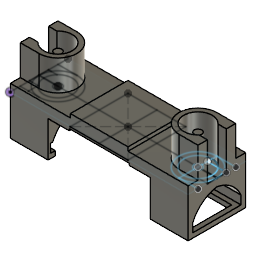
hexbug_cage_final (Autodesk Fusion 360 design; units mm, degrees)
Autodesk Fusion 360 part; units mm, degrees
note: some values were not read from the file. Set by a fixed rule: which sketch regions a step uses.
sketch "Sketch1" plane through (0, 0, 0) normal (0, 0, 1) x (1, 0, 0)
  line L0 (0, 0) -> (46.99, 0)
  line L1 (46.99, 0) -> (46.99, 15.24)
  line L2 (46.99, 15.24) -> (0, 15.24)
  line L3 (0, 15.24) -> (0, 0)
  line L4 (0, 0) -> (0, 1.25)
  line L5 (0, 1.25) -> (46.99, 1.25)
  line L6 (0, 15.24) -> (0, 13.99)
  line L7 (0, 13.99) -> (46.99, 13.99)
  dimension "d1" = 46.99
  dimension "d2" = 15.24
  dimension "d3" = 1.25
  dimension "d4" = 1.25
  constraint horizontal L0
  constraint vertical L1
  constraint horizontal L2
  constraint vertical L3
  constraint coincident L0.start L3.end
  constraint perpendicular L0 L4
  constraint coincident L1 L5.end
  constraint perpendicular L1 L5
  constraint perpendicular L2 L6
  constraint coincident L1 L7.end
  constraint perpendicular L1 L7
  measures "d1" distance of L0.start L0.end
  measures "d2" distance of L0.start L2.end
  measures "d3" distance of L0.start L4.end
  measures "d4" distance of L2.end L6.end
extrude "Extrude1" add sketch "Sketch1" along normal blind 2.27 contours L0 L1 L3 L4 L5 | L1 L2 L3 L6 L7 makes body 1 at (15.6633, 1.25, 0.7567) makes body 2 at (31.3267, 15.24, 0.7567)
sketch "Sketch2" plane through (0, 0, 2.27) normal (0, 0, 1) x (-1, 0, 0)
  line L0 (0, -13.99) -> (-46.99, -13.99)
  line L1 (-46.99, -13.99) -> (-46.99, -15.24)
  line L2 (-46.99, -15.24) -> (0, -15.24)
  line L3 (0, -15.24) -> (0, -13.99)
  line L4 (0, 0) -> (-46.99, 0)
  line L5 (-46.99, 0) -> (-46.99, -15.24)
  line L6 (-46.99, -15.24) -> (0, -15.24)
  line L7 (0, -15.24) -> (0, 0)
  constraint horizontal L4
  constraint vertical L5
  constraint horizontal L6
  constraint vertical L7
  constraint coincident L1.end L2.start
  constraint coincident L4.start L7.end
extrude "Extrude2" add sketch "Sketch2" along normal blind 7.08 contours L0 L4 L5 L7 bodies 1 2
extrude "Extrude3" add 1 faces at (15.6633, 14.8233, 2.27) along direction (0, 0, 1) blind 7.08 on bodies 1 bodies 1
sketch "Sketch3" plane through (0, 0, 0) normal (-1, 0, 0) x (0, -1, 0)
  line L0 (-15.24, 0) -> (-13.99, 0)
  line L1 (-13.99, 0) -> (-13.99, 2.27)
  line L2 (-13.99, 2.27) -> (-1.25, 2.27)
  line L3 (-1.25, 2.27) -> (-1.25, 0)
  line L4 (-1.25, 0) -> (0, 0)
  line L5 (0, 0) -> (0, 9.35)
  line L6 (0, 9.35) -> (-15.24, 9.35)
  line L7 (-15.24, 9.35) -> (-15.24, 0)
  line L8 (-15.24, 2.27) -> (-7.62, 2.27)
  line L9 (-7.62, 2.27) -> (-7.62, 7.35)
  line L10 (-7.62, 7.35) -> (-1.25, 2.27)
  line L11 (-7.62, 7.35) -> (-13.99, 2.27)
  line L12 (-4.435, 4.81) -> (-4.435, 7.35)
  line L13 (-4.435, 7.35) -> (-10.805, 7.35)
  line L14 (-10.805, 7.35) -> (-10.805, 4.81)
  arc A0 (-7.62, 7.35) -> (-13.99, 2.27) centre (-6.1125, -1.0741) ccw
  arc A1 (-1.25, 2.27) -> (-7.62, 7.35) centre (-9.128, -1.0747) ccw
  dimension "d11" = 5.08
  constraint coincident L7 L8.start
  constraint midpoint L2 L8.end
  constraint perpendicular L5 L8
  constraint perpendicular L2 L9
  constraint coincident L2.end L3.start
  constraint coincident L1.end L2.start
  constraint midpoint L10 L12.start
  constraint vertical L12
  constraint perpendicular L9 L13
  constraint midpoint L11 L14.end
  constraint perpendicular L13 L14
  measures "d11" distance of L8.end L9.end
extrude "Extrude4" cut sketch "Sketch3" against normal blind 60 contours L2 L8 L9 L11 | L11 L14 A0 | L2 L9 L10 | L11 L14 A0 | L10 L12 A1 | L10 L12 A1 bodies 1
sketch "Sketch4" plane through (0, 0, 9.35) normal (0, 0, 1) x (-1, 0, 0)
  line L0 (0, 0) -> (-46.99, 0)
  line L1 (-46.99, 0) -> (-46.99, -15.24)
  line L2 (-46.99, -15.24) -> (0, -15.24)
  line L3 (0, -15.24) -> (0, 0)
  line L4 (-46.99, -7.62) -> (0, -7.62)
  line L5 (0, 0) -> (0, -15.24)
  line L6 (0, -7.62) -> (-5, -7.62)
  circle A0 centre (-5, -7.62) radius 1
  line L7 (-46.99, -7.62) -> (-41.99, -7.62)
  circle A1 centre (-41.99, -7.62) radius 1
  line L8 (-41.99, -7.62) -> (-41.99, -8.62)
  line L9 (-41.99, -7.62) -> (-41.99, -6.62)
  circle A2 centre (-41.99, -7.62) radius 5
  line L10 (-41.99, -10.12) -> (-46.99, -10.12)
  circle A3 centre (-41.99, -7.62) radius 3.75
  circle A4 centre (-5, -7.62) radius 3.75
  circle A5 centre (-5, -7.62) radius 5
  line L11 (-23.495, -7.62) -> (-23.495, -15.24)
  line L12 (-23.495, -7.62) -> (-23.495, 0)
  line L13 (-15.875, -15.24) -> (-31.115, -15.24)
  line L14 (-31.115, -15.24) -> (-31.115, 0)
  line L15 (-31.115, 0) -> (-15.875, 0)
  line L16 (-15.875, 0) -> (-15.875, -15.24)
  line L17 (-15.875, -15.24) -> (-31.115, 0) construction
  line L18 (-31.115, -15.24) -> (-15.875, 0) construction
  line L19 (0, -7.62) -> (0, -5.12)
  line L20 (0, -5.12) -> (-0.6699, -5.12)
  line L21 (0, -7.62) -> (0, -10.12)
  line L22 (0, -10.12) -> (-0.6699, -10.12)
  line L23 (0, -10.12) -> (-2.2049, -10.12)
  line L24 (0, -5.12) -> (-2.2049, -5.12)
  line L25 (-2.2049, -5.12) -> (-2.2049, -2.62)
  line L26 (-2.2049, -2.62) -> (-5, -2.62)
  line L27 (-2.2049, -2.62) -> (0, -2.62)
  line L28 (-5, -12.62) -> (0, -12.62)
  line L29 (-41.99, -7.62) -> (-41.99, -2.62)
  line L30 (-41.99, -2.62) -> (-46.99, -2.62)
  line L31 (-46.99, -7.62) -> (-46.99, -5.12)
  line L32 (-46.99, -5.12) -> (-44.7851, -5.12)
  line L33 (-46.99, -7.62) -> (-46.99, -10.12)
  line L34 (-46.99, -10.12) -> (-44.7851, -10.12)
  line L35 (-41.99, -7.62) -> (-41.99, -12.62)
  line L36 (-41.99, -12.62) -> (-46.99, -12.62)
  point P0 (-23.495, -7.62)
  dimension "d14" = 5
  dimension "d15" = 2
  dimension "d17" = 2
  dimension "d29" = 10
  dimension "d30" = 7.5
  dimension "d35" = 7.5
  dimension "d36" = 10
  dimension "d41" = 15.24
  dimension "d42" = 15.24
  dimension "d45" = 5
  dimension "d46" = 2.5
  dimension "d47" = 2.5
  dimension "d52" = 2.5
  dimension "d55" = 2.5
  dimension "d56" = 2.5
  constraint midpoint L1 L4.start
  constraint midpoint L3 L4.end
  constraint coincident L0.start L3.end
  constraint coincident L2.end L3.start
  constraint perpendicular L5 L6
  constraint coincident L6.end A0.centre
  constraint perpendicular L1 L7
  constraint coincident L7.end A1.centre
  constraint coincident A1 L8.end
  constraint perpendicular L4 L8
  constraint coincident A1 L9.end
  constraint perpendicular L7 L9
  constraint coincident L1 L10.end
  constraint perpendicular L1 L10
  constraint concentric A2 A3
  constraint concentric A0 A4
  constraint concentric A4 A5
  constraint midpoint L4 P0
  constraint midpoint L2 L11.end
  constraint midpoint L0 L12.end
  constraint horizontal L13
  constraint perpendicular L13 L14
  constraint parallel L13 L15
  constraint parallel L14 L16
  constraint coincident L17 P0
  constraint coincident L18 P0
  constraint coincident L2 L13.start
  constraint coincident P0 L11.start
  constraint coincident A5 L4.end
  constraint coincident L4 L6.start
  constraint perpendicular L4 L19
  constraint coincident A5 L20.end
  constraint perpendicular L19 L20
  constraint perpendicular L4 L21
  constraint coincident A5 L22.end
  constraint perpendicular L21 L22
  constraint coincident A4 L23.end
  constraint perpendicular L21 L23
  constraint coincident A4 L24.end
  constraint perpendicular L19 L24
  constraint perpendicular L24 L25
  constraint coincident A5 L26.end
  constraint tangent A5 L26
  constraint coincident L5 L27.end
  constraint perpendicular L5 L27
  constraint coincident A5 L28.start
  constraint coincident L5 L28.end
  constraint tangent A5 L28
  constraint perpendicular L5 L28
  constraint coincident A2 L29.end
  constraint parallel L9 L29
  constraint coincident L1 L30.end
  constraint tangent A2 L30
  constraint perpendicular L4 L31
  constraint coincident A3 L32.end
  constraint perpendicular L31 L32
  constraint perpendicular L32 L33
  constraint coincident L10 L34.end
  constraint coincident A3 L34.end
  constraint coincident A2 L35.end
  constraint vertical L35
  constraint coincident L1 L36.end
  constraint tangent A2 L36
  measures "d14" distance of L4.end L6.end
  measures "d17" diameter of A1
  measures "d29" diameter of A2
  measures "d30" diameter of A3
  measures "d41" distance of L14.end L15.end
  measures "d42" distance of L13.end L14.end
  measures "d45" distance of L10.start L10.end
  measures "d46" distance of L4.end L19.end
  measures "d47" distance of L4.end L21.end
  measures "d52" distance of L24.end L25.end
  measures "d55" distance of L4.start L31.end
  measures "d56" distance of L4.start L10.end
extrude "Extrude6" add sketch "Sketch4" along normal blind 8 contours L4 A1 L8 L35 | L4 A1 L9 L29 | L4 L7 A1 L9 L29 | L4 L7 A1 L8 L35 bodies 1
extrude "Extrude9" add sketch "Sketch4" along normal blind 8 contours L4 L6 A0 | L4 L6 A0 bodies 1
extrude "Extrude11" add sketch "Sketch4" along normal blind 2 contours L0 L4 L12 L15 L16 | L0 L4 L12 L14 L15 | L2 L4 L11 L13 L16 | L2 L4 L11 L13 L14 bodies 1
extrude "Extrude14" add sketch "Sketch4" along normal blind 10 contours L3 L5 A5 L20 L24 L25 L27 | A5 L25 L26 | L4 A4 A5 L25 | L4 A4 A5 L23 | A5 L24 L25 | L3 L5 A5 L22 L23 L28 bodies 1
extrude "Extrude15" add sketch "Sketch4" along normal blind 10 contours L1 A2 L30 L32 | L4 A2 A3 L35 | L4 A2 A3 L29 | A2 A3 L29 L32 | L1 A2 L10 L34 L36 | A2 L10 A3 L34 L35 bodies 1
sketch "Sketch5" plane through (0, 0, 0) normal (0, 1, 0) x (1, 0, 0)
  line L0 (0, 0) -> (46.99, 0)
  line L1 (23.495, 0) -> (23.495, -7.25)
  line L2 (0, 0) -> (10, 0)
  line L3 (46.99, 0) -> (36.99, 0)
  line L4 (36.99, 0) -> (36.99, -7.25)
  line L5 (10, 0) -> (10, -9.25)
  line L6 (23.495, 0) -> (28.495, 0)
  line L7 (23.495, 0) -> (18.495, 0)
  line L8 (28.495, 0) -> (28.495, -9.25)
  line L9 (0, 0) -> (0, -9.25)
  line L10 (0, -9.25) -> (46.99, -9.25)
  line L11 (46.99, -9.25) -> (46.99, 0)
  line L12 (23.495, 0) -> (18.495, 0)
  line L13 (18.495, 0) -> (18.495, -9.25)
  line L14 (23.495, -7.25) -> (46.99, -7.25)
  line L15 (23.495, -7.25) -> (0, -7.25)
  dimension "d59" = 46.99
  dimension "d60" = 7.25
  dimension "d61" = 10
  dimension "d62" = 10
  dimension "d63" = 7.25
  dimension "d64" = 9.25
  dimension "d65" = 5
  dimension "d66" = 5
  dimension "d67" = 9.25
  dimension "d68" = 9.25
  dimension "d69" = 46.99
  constraint coincident L0.start L2.start
  constraint horizontal L0
  constraint midpoint L0 L1.start
  constraint perpendicular L0 L1
  constraint parallel L0 L2
  constraint parallel L0 L3
  constraint perpendicular L3 L4
  constraint perpendicular L2 L5
  constraint perpendicular L1 L6
  constraint perpendicular L1 L7
  constraint perpendicular L6 L8
  constraint perpendicular L2 L9
  constraint perpendicular L4 L10
  constraint coincident L10 L13.end
  constraint perpendicular L10 L13
  constraint coincident L11 L14.end
  constraint perpendicular L11 L14
  constraint coincident L9 L15.end
  constraint perpendicular L9 L15
  measures "d59" distance of L0.start L0.end
  measures "d60" distance of L1.start L1.end
  measures "d61" distance of L0.start L2.end
  measures "d62" distance of L0.end L3.end
  measures "d63" distance of L3.end L4.end
  measures "d64" distance of L2.end L5.end
  measures "d65" distance of L1.start L6.end
  measures "d66" distance of L1.start L7.end
  measures "d67" distance of L6.end L8.end
  measures "d68" distance of L0.start L9.end
  measures "d69" distance of L9.end L10.end
extrude "Extrude16" cut sketch "Sketch5" along normal blind 50 contours L0 L5 L13 L15 | L0 L1 L7 L12 L13 L15 | L0 L1 L6 L8 L14 | L0 L4 L8 L14 bodies 1
sketch "Sketch6" plane through (0, 0, 9.35) normal (0, 0, 1) x (-1, 0, 0)
  line L0 (0, 0) -> (0, -15.24)
  line L1 (0, 0) -> (-1.25, 0)
  line L2 (0, -15.24) -> (-1.25, -15.24)
  line L3 (-1.25, -15.24) -> (-1.25, 0)
  line L4 (-1.25, 0) -> (0, 0)
  line L5 (0, 0) -> (0, -15.24)
  dimension "d72" = 15.24
  dimension "d73" = 1.25
  constraint coincident L0.start L1.start
  constraint vertical L0
  constraint perpendicular L0 L1
  constraint horizontal L2
  constraint vertical L3
  constraint horizontal L4
  constraint vertical L5
  measures "d72" distance of L0.start L0.end
  measures "d73" distance of L0.start L1.end
extrude "Extrude17" add sketch "Sketch6" against normal blind 9.35 bodies 1
sketch "Sketch7" plane through (46.99, 0, 0) normal (1, 0, 0) x (0, 1, 0)
  arc A0 (7.62, 7.35) -> (1.25, 2.27) centre (9.128, -1.0747) ccw
  arc A1 (13.99, 2.27) -> (7.62, 7.35) centre (6.1125, -1.0741) ccw
  line L0 (13.99, 2.27) -> (13.99, 0)
  line L1 (13.99, 0) -> (15.24, 0)
  line L2 (15.24, 0) -> (15.24, 9.35)
  line L3 (15.24, 9.35) -> (12.62, 9.35)
  line L4 (12.62, 9.35) -> (12.62, 19.35)
  line L5 (12.62, 19.35) -> (10.12, 19.35)
  line L6 (10.12, 19.35) -> (10.12, 9.35)
  line L7 (10.12, 9.35) -> (5.12, 9.35)
  line L8 (5.12, 9.35) -> (5.12, 19.35)
  line L9 (5.12, 19.35) -> (2.62, 19.35)
  line L10 (2.62, 19.35) -> (2.62, 9.35)
  line L11 (2.62, 9.35) -> (0, 9.35)
  line L12 (0, 9.35) -> (0, 0)
  line L13 (0, 0) -> (1.25, 0)
  line L14 (1.25, 0) -> (1.25, 2.27)
  line L15 (0, 9.35) -> (15.24, 9.35)
  line L16 (15.24, 9.35) -> (15.24, 0)
  line L17 (15.24, 0) -> (0, 0)
  line L18 (0, 0) -> (0, 9.35)
  constraint horizontal L15
  constraint vertical L16
  constraint horizontal L17
  constraint vertical L18
  constraint coincident L1.end L2.start
  constraint coincident L11.end L12.start
extrude "Extrude18" add sketch "Sketch7" along normal blind 1.25 contours A0 A1 L0 L14 L17 | A0 A1 L0 L1 L2 L3 L7 L11 L12 L13 L14 L15 L16 L17 L18 bodies 1
extrude "Extrude19" add 1 faces at (47.8233, 5.4967, 0) along direction (0, 0, -1) blind 1.25 on bodies 1 bodies 1
sketch "Sketch8" plane through (46.99, 0, 0) normal (-1, 0, 0) x (0, -1, 0)
  line L0 (-1.25, -1.25) -> (-1.25, 2.27)
  arc A0 (-1.25, 2.27) -> (-7.62, 7.35) centre (-9.128, -1.0747) ccw
  arc A1 (-7.62, 7.35) -> (-13.99, 2.27) centre (-6.1125, -1.0741) ccw
  line L1 (-13.99, 2.27) -> (-13.99, -1.25)
  line L2 (-13.99, -1.25) -> (-1.25, -1.25)
  line L3 (-1.25, -1.25) -> (-13.99, -1.25)
  line L4 (-13.99, -1.25) -> (-13.99, 0)
  line L5 (-13.99, 0) -> (-1.25, 0)
  line L6 (-1.25, 0) -> (-1.25, -1.25)
  dimension "d80" = 1.25
  constraint coincident L0.start L2.end
  constraint coincident L1.end L2.start
  constraint perpendicular L3 L4
  constraint coincident L0 L5.end
  constraint perpendicular L0 L5
  measures "d80" distance of L1.end L4.end
extrude "Extrude20" add sketch "Sketch8" along normal blind 1.25 contours L0 L1 L2 L3 L4 L5 L6 bodies 1
sketch "Sketch9" plane through (0, 1.25, 0) normal (0, 1, 0) x (-1, 0, 0)
  line L0 (-46.99, 0) -> (-45.74, 0)
  line L1 (-45.74, 0) -> (-45.74, -1.25)
  line L2 (-45.74, -1.25) -> (-36.99, -1.25)
  line L3 (-36.99, -1.25) -> (-36.99, 2.27)
  line L4 (-36.99, 2.27) -> (-46.99, 2.27)
  line L5 (-46.99, 2.27) -> (-46.99, 0)
  line L6 (-45.74, 0) -> (-36.99, 0)
  line L7 (-36.99, 0) -> (-36.99, -1.25)
  line L8 (-36.99, -1.25) -> (-45.74, -1.25)
  constraint coincident L0.end L1.start
  constraint coincident L3 L6.end
  constraint perpendicular L3 L6
  constraint coincident L2.end L3.start
  constraint coincident L1.end L2.start
extrude "Extrude21" add sketch "Sketch9" along normal blind 1.25 contours L1 L2 L3 L6 L7 L8 bodies 1
sketch "Sketch10" plane through (0, 13.99, 0) normal (0, -1, 0) x (1, 0, 0)
  line L0 (45.74, -1.25) -> (45.74, 0)
  line L1 (45.74, 0) -> (46.99, 0)
  line L2 (46.99, 0) -> (46.99, 2.27)
  line L3 (46.99, 2.27) -> (36.99, 2.27)
  line L4 (36.99, 2.27) -> (36.99, -1.25)
  line L5 (36.99, -1.25) -> (45.74, -1.25)
  line L6 (45.74, 0) -> (36.99, 0)
  line L7 (36.99, 0) -> (36.99, -1.25)
  line L8 (36.99, -1.25) -> (45.74, -1.25)
  constraint coincident L0.end L1.start
  constraint coincident L4 L6.end
  constraint perpendicular L4 L6
  constraint coincident L4.end L5.start
  constraint coincident L0.start L5.end
extrude "Extrude22" add sketch "Sketch10" along normal blind 1.25 contours L0 L4 L5 L6 L7 L8 bodies 1
extrude "Extrude23" cut 1 faces at (48.24, 10.16, 2.2833) along direction (-1, 0, 0) blind 1.25 on bodies 1 bodies 1
extrude "Extrude24" cut 1 faces at (4.1667, 1.25, 0.7567) along direction (0, -1, 0) blind 0.2 on bodies 1 bodies 1
extrude "Extrude25" cut 1 faces at (4.1667, 13.99, 0.7567) along direction (0, 1, 0) blind 0.2 on bodies 1 bodies 1
sketch "Sketch11" plane through (0, 0, 7.25) normal (0, 0, -1) x (1, 0, 0)
  line L0 (36.99, -8.0993) -> (10, -8.0993)
  line L1 (10, -8.0993) -> (10, -15.24)
  line L2 (10, -15.24) -> (36.99, -15.24)
  line L3 (36.99, -15.24) -> (36.99, -8.0993)
  line L4 (23.495, -15.24) -> (23.495, 0)
  line L5 (23.495, -15.24) -> (15.595, -15.24)
  line L6 (15.595, -15.24) -> (15.595, 0)
  line L7 (15.595, 0) -> (23.495, 0)
  line L8 (23.495, 0) -> (23.495, -15.24)
  line L9 (23.495, -15.24) -> (31.395, -15.24)
  line L10 (31.395, -15.24) -> (31.395, 0)
  line L11 (31.395, 0) -> (23.495, 0)
  line L12 (23.495, 0) -> (23.495, -15.24)
  dimension "d93" = 15.24
  dimension "d94" = 15.24
  dimension "d95" = 7.9
  dimension "d96" = 7.9
  constraint midpoint L2 L4.start
  constraint perpendicular L0 L4
  constraint horizontal L5
  constraint vertical L6
  constraint horizontal L7
  constraint vertical L8
  constraint horizontal L9
  constraint vertical L10
  constraint horizontal L11
  constraint vertical L12
  measures "d93" distance of L4.start L4.end
  measures "d94" distance of L4.start L4.end
  measures "d95" distance of L6.end L4.end
  measures "d96" distance of L10.end L4.end
extrude "Extrude26" cut sketch "Sketch11" against normal blind 1.5 contours L0 L2 L4 L8 L9 L10 L12 | L0 L4 L8 L10 L11 L12 | L0 L2 L4 L5 L6 L8 L12 | L0 L4 L6 L7 L8 L12 bodies 1
extrude "Extrude27" cut 1 faces at (4.1667, 14.19, 0.7567) along direction (0, 1, 0) blind 0.2 on bodies 1 bodies 1
extrude "Extrude28" cut 1 faces at (4.1667, 1.05, 0.7567) along direction (0, -1, 0) blind 0.2 on bodies 1 bodies 1
extrude "Extrude29" cut 2 faces at (13.73, 4.7605, 7.25) (11.865, 10.4795, 7.25) along direction (0, 0, 1) blind 1 on bodies 1 bodies 1
extrude "Extrude30" cut 1 faces at (11.865, 8.0993, 7.5833) along direction (0, -1, 0) blind 10 on bodies 1 bodies 1
extrude "Extrude31" cut 2 faces at (35.125, 2.3803, 7.25) (35.125, 10.4795, 7.25) along direction (0, 0, 1) blind 1 on bodies 1 bodies 1
extrude "Extrude32" cut 1 faces at (33.26, 7.1408, 7.9167) along direction (0, 1, 0) blind 10 on bodies 1 bodies 1
extrude "Extrude33" add 1 faces at (31.115, 10.16, 10.0167) along direction (1, 0, 0) blind 5 on bodies 1 bodies 1
extrude "Extrude34" add 1 faces at (15.875, 5.08, 10.0167) along direction (-1, 0, 0) blind 5 on bodies 1 bodies 1
sketch "Sketch12" plane through (0, 0, 11.35) normal (0, 0, 1) x (-1, 0, 0)
  line L0 (-10.875, 0) -> (-36.115, 0)
  line L1 (-36.115, 0) -> (-36.115, -15.24)
  line L2 (-36.115, -15.24) -> (-10.875, -15.24)
  line L3 (-10.875, -15.24) -> (-10.875, 0)
  line L4 (-23.495, -15.24) -> (-23.495, 0)
  line L5 (-23.495, -7.62) -> (-31.115, -7.62)
  line L6 (-23.495, -7.62) -> (-15.875, -7.62)
  line L7 (-31.115, -7.62) -> (-31.115, 0)
  line L8 (-31.115, 0) -> (-23.495, 0)
  line L9 (-15.875, -7.62) -> (-15.875, -15.24)
  line L10 (-15.875, -15.24) -> (-31.115, -15.24)
  line L11 (-31.115, -15.24) -> (-31.115, 0)
  line L12 (-31.115, 0) -> (-15.875, 0)
  line L13 (-15.875, 0) -> (-15.875, -15.24)
  dimension "d115" = 7.62
  dimension "d116" = 7.62
  constraint midpoint L2 L4.start
  constraint midpoint L0 L4.end
  constraint midpoint L4 L5.start
  constraint perpendicular L4 L5
  constraint perpendicular L4 L6
  constraint coincident L0 L7.end
  constraint perpendicular L0 L7
  constraint coincident L2 L9.end
  constraint perpendicular L2 L9
  constraint horizontal L10
  constraint vertical L11
  constraint horizontal L12
  constraint vertical L13
  measures "d115" distance of L5.start L5.end
  measures "d116" distance of L5.start L6.end
extrude "Extrude35" add sketch "Sketch12" along normal blind 1 contours L0 L4 L6 L12 L13 | L0 L4 L5 L7 L8 L11 L12 | L2 L4 L6 L9 L10 L13 | L2 L4 L5 L10 L11 bodies 1
extrude "Extrude36" add 1 faces at (36.115, 10.16, 10.0167) along direction (1, 0, 0) blind 0.87 on bodies 1 bodies 1
extrude "Extrude37" add 1 faces at (10.875, 5.08, 10.0167) along direction (-1, 0, 0) blind 0.87 on bodies 1 bodies 1
extrude "Extrude38" add sketch "Sketch4" along normal blind 2 contours L0 L3 L4 L5 A5 L16 L26 L27 bodies 1
extrude "Extrude39" add 1 faces at (5.0017, 14.3667, 9.35) along direction (0, 0, 1) blind 2 on bodies 1 bodies 1
extrude "Extrude40" add 1 faces at (41.9883, 14.3667, 9.35) along direction (0, 0, 1) blind 2 on bodies 1 bodies 1
extrude "Extrude41" add 1 faces at (0.4167, 5.3633, 0) along direction (0, 0, -1) blind 1.25 on bodies 1 bodies 1
sketch "Sketch13" plane through (1.25, 0, 0) normal (1, 0, 0) x (0, 1, 0)
  line L0 (14.39, -1.25) -> (14.39, 2.27)
  line L1 (14.39, 2.27) -> (13.99, 2.27)
  arc A0 (13.99, 2.27) -> (7.62, 7.35) centre (6.1125, -1.0741) ccw
  arc A1 (7.62, 7.35) -> (1.25, 2.27) centre (9.128, -1.0747) ccw
  line L2 (1.25, 2.27) -> (0.85, 2.27)
  line L3 (0.85, 2.27) -> (0.85, -1.25)
  line L4 (0.85, -1.25) -> (14.39, -1.25)
  line L5 (0.85, -1.25) -> (14.39, -1.25)
  line L6 (14.39, -1.25) -> (14.39, 0)
  line L7 (14.39, 0) -> (0.85, 0)
  line L8 (0.85, 0) -> (0.85, -1.25)
  dimension "d131" = 1.25
  constraint horizontal L5
  constraint vertical L6
  constraint horizontal L7
  constraint vertical L8
  constraint coincident L3.end L4.start
  measures "d131" distance of L3.end L7.end
extrude "Extrude42" add sketch "Sketch13" along normal blind 1.25 contours L0 L3 L4 L5 L6 L7 L8 bodies 1
extrude "Extrude43" cut 1 faces at (7.5, 14.39, 0.34) along direction (0, 1, 0) blind 0.2 on bodies 1 bodies 1
extrude "Extrude44" cut 1 faces at (7.5, 0.85, 0.34) along direction (0, -1, 0) blind 0.2 on bodies 1 bodies 1
sketch "Sketch14" plane through (0, 0.65, 0) normal (0, 1, 0) x (-1, 0, 0)
  line L0 (-2.5, 0) -> (-1.25, 0)
  line L1 (-1.25, 0) -> (-1.25, 2.27)
  line L2 (-1.25, 2.27) -> (-10, 2.27)
  line L3 (-10, 2.27) -> (-10, -1.25)
  line L4 (-10, -1.25) -> (-2.5, -1.25)
  line L5 (-2.5, -1.25) -> (-2.5, 0)
  line L6 (-2.5, 0) -> (-10, 0)
  line L7 (-10, 0) -> (-10, -1.25)
  line L8 (-10, -1.25) -> (-2.5, -1.25)
  line L9 (-2.5, -1.25) -> (-2.5, 0)
  constraint horizontal L6
  constraint vertical L7
  constraint horizontal L8
  constraint vertical L9
  constraint coincident L3.end L4.start
  constraint coincident L0.start L5.end
extrude "Extrude45" add sketch "Sketch14" along normal blind 1.25 contours L3 L4 L5 L6 L7 L8 L9 bodies 1
sketch "Sketch15" plane through (0, 14.59, 0) normal (0, -1, 0) x (1, 0, 0)
  line L0 (2.5, 0) -> (2.5, -1.25)
  line L1 (2.5, -1.25) -> (10, -1.25)
  line L2 (10, -1.25) -> (10, 2.27)
  line L3 (10, 2.27) -> (1.25, 2.27)
  line L4 (1.25, 2.27) -> (1.25, 0)
  line L5 (1.25, 0) -> (2.5, 0)
  line L6 (2.5, 0) -> (10, 0)
  line L7 (10, 0) -> (10, -1.25)
  line L8 (10, -1.25) -> (2.5, -1.25)
  line L9 (2.5, -1.25) -> (2.5, 0)
  constraint horizontal L6
  constraint vertical L7
  constraint horizontal L8
  constraint vertical L9
  constraint coincident L1.end L2.start
  constraint coincident L0.start L5.end
extrude "Extrude46" add sketch "Sketch15" along normal blind 1.25 contours L0 L1 L2 L6 L7 L8 L9 bodies 1
extrude "Extrude12" [suppressed]
equation "d115 = ( 1.524 / 2 ) * 1 cm"
